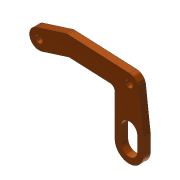
# Autodesk Inventor part: COXA_YAW_SUPPORT-LINK_BACK
Saved by Autodesk Inventor 2019.4 (Build 234330000, 330)
## iProperties
Created: 2019-10-21
Part Number: COXA_YAW_SUPPORT-LINK_BACK
Material: 一般
Document SubType Name: Modeling
Designer: y6tada
Density: 1 g/cm^3
Appearance: 滑らか - 淡いオレンジ
Author: y6tada
Autodesk Inventor part; units mm, degrees
ref_plane "YZ Plane" through (0, 0, 0) normal (1, 0, 0) x (0, 1, 0)
ref_plane "XZ Plane" through (0, 0, 0) normal (0, 1, 0) x (-1, 0, 0)
ref_plane "XY Plane" through (0, 0, 0) normal (0, 0, 1) x (1, 0, 0)
sketch "スケッチ1" plane through (0, 0, 0) normal (0, 0, 1) x (1, 0, 0)
  line L0 (0, 0) -> (0, -20) construction
  line L1 (0, -20) -> (-37.9074, -2.6507) construction
  line L2 (-37.9074, -2.6507) -> (0, 0) construction
  arc A0 (-39.115, 1.1626) -> (-36.6999, -6.4641) centre (-37.9074, -2.6507) ccw
  arc A1 (3.9565, 0.5882) -> (0.1846, 3.9957) centre (0, 0) ccw
  arc A2 (-6.5, -23) -> (6.5, -23) centre (0, -23) ccw
  arc A3 (3.5, -17) -> (-3.5, -17) centre (0, -17) ccw
  arc A4 (-3.5, -23) -> (3.5, -23) centre (0, -23) ccw
  line L3 (-3.5, -17) -> (-3.5, -23)
  line L4 (3.5, -17) -> (3.5, -23)
  line L5 (0, -23) -> (0, -17) construction
  line L6 (3.9565, 0.5882) -> (6.4293, -16.0441)
  line L7 (6.5, -17) -> (6.5, -23)
  arc A5 (6.5, -17) -> (6.4293, -16.0441) centre (0, -17) ccw
  line L8 (-39.115, 1.1626) -> (-26.8131, 5.0582)
  line L9 (-25.769, 5.1949) -> (0.1846, 3.9957)
  arc A6 (-25.769, 5.1949) -> (-26.8131, 5.0582) centre (-25.9074, 2.1981) ccw
  line L10 (-37.9074, -2.6507) -> (-25.9074, 2.1981) construction
  line L11 (-6.5, -23) -> (-6.5, -5.6137)
  line L12 (-25.2478, -2.8377) -> (-36.6999, -6.4641)
  line L13 (-25.2478, -2.8377) -> (-8.4077, -3.6158)
  arc A7 (-6.5, -5.6137) -> (-8.4077, -3.6158) centre (-8.5, -5.6137) ccw
  dimension "d0" = 20
  dimension "d2" = 38
  dimension "d3" = 4
  dimension "d13" = 6
  dimension "d14" = 3.5
  dimension "d15" = 6.5
  dimension "d17" = 3
  dimension "d18" = 4
  dimension "d20" = 12
  dimension "d21" = 86
  dimension "d22" = 8
  dimension "d23" = 2
  constraints: 28 end point, 18 point on circle, 16 tangent, 8 centre point, 6 coincident, 3 point on line, 3 vertical, 2 concentric, 2 equal radius, 2 parallel, 1 midpoint
  measures "d0" distance of L0.end L0.start
  measures "d2" distance of L1.end L0.start
  measures "d3" radius of A0
  measures "d13" distance of L5.start L5.end
  measures "d14" radius of A3
  measures "d15" radius of A2
  measures "d17" radius of A6
  measures "d18" distance from line of L10.end L2
  measures "d20" horizontal distance of L10.start L10.end
  measures "d21" angle of L0 L2
  measures "d22" distance between parallel lines of L13 L9
  measures "d23" radius of A7
extrude "押し出し1" add sketch "スケッチ1" along normal blind 3
hole "穴1" at (-37.9074, -2.6507, 0) at (0, 0, 0) direction (0, 0, 1) diameter 3 end through all
sketch "スケッチ2" plane through (0, 0, 3) normal (0, 0, 1) x (1, 0, 0)
  arc A0 (3.5, -17) -> (-3.5, -17) centre (0, -17) ccw projected
  line L0 (3.5, -17) -> (3.5, -23) projected
  arc A1 (-3.5, -23) -> (3.5, -23) centre (0, -23) ccw projected
  line L1 (-3.5, -23) -> (-3.5, -17) projected
  point P0 (0, 0)
extrude "押し出し2" add sketch "スケッチ2" against normal blind 0.4
